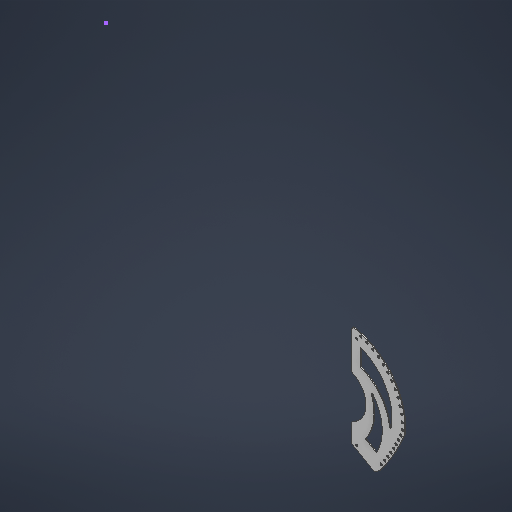
# Autodesk Inventor part: TopCurve
Saved by Autodesk Inventor 2026.1 (Build 301233000, 233)
## iProperties
Created: 2026-03-09
Part Number: TopCurve
Material: Generic
Document SubType Name: Modeling
Designer: roejo
Density: 1 g/cm^3
Appearance: Default
Author: roejo
Autodesk Inventor part; units mm, degrees
ref_plane "YZ Plane" through (0, 0, 0) normal (1, 0, 0) x (0, 1, 0)
ref_plane "XZ Plane" through (0, 0, 0) normal (0, 1, 0) x (-1, 0, 0)
ref_plane "XY Plane" through (0, 0, 0) normal (0, 0, 1) x (1, 0, 0)
sketch "Sketch1" plane through (0, 0, 0) normal (0, 0, 1) x (1, 0, 0)
  circle A0 centre (241.6154, -140.1465) radius 2.4638
  arc A1 (259.0779, -181.0227) -> (259.0779, -99.2703) centre (241.6154, -140.1465) ccw
  line L0 (259.0779, -218.2466) -> (259.0779, -181.0227)
  arc A2 (312.3724, -235.9031) -> (359.2204, -154.9095) centre (11.2573, -7.6879) ccw
  arc A3 (359.2204, -154.9095) -> (360.17, -151.1328) centre (347.5241, -149.9609) ccw
  arc A4 (360.17, -151.1328) -> (262.8183, -22.9871) centre (241.6154, -140.1465) ccw
  arc A5 (301.8563, -242.8447) -> (312.3724, -235.9031) centre (241.6154, -140.1465) ccw
  arc A6 (262.8183, -22.9871) -> (259.0779, -26.1114) centre (262.2529, -26.1114) ccw
  line L1 (259.0779, -26.1114) -> (259.0779, -99.2703)
  line L2 (259.0779, -181.0227) -> (259.0779, -218.2466)
  circle A7 centre (268.2854, -38.5465) radius 2.1844
  circle A8 centre (268.2854, -216.3465) radius 2.1844
  arc A9 (308.9934, -232.4758) -> (354.8343, -153.0538) centre (11.2573, -7.6879) ccw
  arc A10 (354.8343, -153.0538) -> (355.4278, -150.6933) centre (347.5241, -149.9609) ccw
  arc A11 (355.4278, -150.6933) -> (263.8404, -28.0281) centre (241.6154, -140.1465) ccw
  circle A12 centre (263.8404, -28.0281) radius 2.413
  circle A13 centre (276.0241, -31.1486) radius 2.413
  circle A14 centre (287.7911, -35.5889) radius 2.413
  circle A15 centre (298.9991, -41.2951) radius 2.413
  circle A16 centre (309.5123, -48.1981) radius 2.413
  circle A17 centre (319.2034, -56.2144) radius 2.413
  circle A18 centre (327.9551, -65.247) radius 2.413
  circle A19 centre (335.6615, -75.1863) radius 2.413
  circle A20 centre (342.2292, -85.9122) radius 2.413
  circle A21 centre (347.5787, -97.2948) radius 2.413
  circle A22 centre (351.6452, -109.1961) radius 2.413
  circle A23 centre (354.3796, -121.4722) radius 2.413
  circle A24 centre (355.7487, -133.9744) radius 2.413
  circle A25 centre (355.7358, -146.5513) radius 2.413
  circle A26 centre (353.0365, -157.2317) radius 2.413
  circle A27 centre (348.7088, -166.7567) radius 2.413
  circle A28 centre (344.0523, -176.2817) radius 2.413
  circle A29 centre (339.0531, -185.8067) radius 2.413
  circle A30 centre (333.6952, -195.3317) radius 2.413
  circle A31 centre (327.9604, -204.8567) radius 2.413
  circle A32 centre (321.8278, -214.3817) radius 2.413
  circle A33 centre (315.2734, -223.9067) radius 2.413
  line L3 (301.8563, -242.8447) -> (259.0779, -218.2466)
  point P0 (259.0779, -22.3716)
  point P1 (295.3179, -246.41)
  dimension "d4" = 88.9
  dimension "d5" = 12.7
  dimension "d7" = 4.3688
  dimension "d8" = 4.7625
  dimension "d9" = 4.826
  dimension "d12" = 82
  dimension "d14" = 4.826
  dimension "d21" = 4.826
  dimension "d22" = 4.826
  dimension "d23" = 4.826
  dimension "d24" = 4.826
  dimension "d25" = 4.826
  dimension "d26" = 4.826
  dimension "d27" = 4.826
  dimension "d28" = 9.525
  dimension "d29" = 9.525
  dimension "d30" = 9.525
  dimension "d31" = 9.525
  dimension "d32" = 9.525
  dimension "d33" = 9.525
  dimension "d34" = 9.525
  dimension "d41" = 177.8
  dimension "d42" = 9.2075
  constraints: 33 centre point, 18 point on circle, 8 end point, 4 tangent, 3 coincident, 45 other
  measures "d4" diameter of A1
  measures "d5" radius of A3
  measures "d7" diameter of A8
  measures "d8" radial gap between concentric circles of A4 A11
  measures "d9" diameter of A12
  measures "d14" diameter of A26
  measures "d21" diameter of A27
  measures "d22" diameter of A28
  measures "d23" diameter of A29
  measures "d24" diameter of A30
  measures "d25" diameter of A31
  measures "d26" diameter of A32
  measures "d27" diameter of A33
  measures "d28" vertical distance of A27.centre A26.centre
  measures "d29" vertical distance of A28.centre A27.centre
  measures "d30" vertical distance of A29.centre A28.centre
  measures "d31" vertical distance of A30.centre A29.centre
  measures "d32" vertical distance of A31.centre A30.centre
  measures "d33" vertical distance of A32.centre A31.centre
  measures "d34" vertical distance of A32.centre A33.centre
  measures "d41" distance of A8.centre A7.centre
  measures "d42" distance from line of L1 A7.centre
extrude "Extrusion1" add sketch "Sketch1" along normal blind 1.5875 contours A1 L1 A6 A4 A3 A2 A5 L3 L0
sketch "Sketch4" plane through (0, 0, 1.5875) normal (0, 0, 1) x (1, 0, 0)
  point P0 (-212.5628, 245.6595)
sketch "Sketch6" plane through (0, 0, 1.5875) normal (0, 0, 1) x (1, 0, 0)
  circle A0 centre (263.8404, -28.0281) radius 2.413 projected
  point P0 (0, 0)
extrude "Extrusion4" add sketch "Sketch6" against normal blind 1.5875
sketch "Sketch7" plane through (0, 0, 1.5875) normal (0, 0, 1) x (1, 0, 0)
  arc A0 (259.0779, -181.0227) -> (259.0779, -99.2703) centre (241.6154, -140.1465) ccw projected
  arc A1 (360.17, -151.1328) -> (262.8183, -22.9871) centre (241.6154, -140.1465) ccw projected
  arc A2 (359.2204, -154.9095) -> (360.17, -151.1328) centre (347.5241, -149.9609) ccw projected
  arc A3 (312.3724, -235.9031) -> (359.2204, -154.9095) centre (11.2573, -7.6879) ccw projected
  arc A4 (301.8563, -242.8447) -> (312.3724, -235.9031) centre (241.6154, -140.1465) ccw projected
  line L0 (259.0779, -218.2466) -> (301.8563, -242.8447) projected
  line L1 (259.0779, -181.0227) -> (259.0779, -218.2466) projected
  line L2 (259.0779, -26.1114) -> (259.0779, -99.2703) projected
  arc A5 (262.8183, -22.9871) -> (259.0779, -26.1114) centre (262.2529, -26.1114) ccw projected
  arc A6 (306.6939, -207.6622) -> (299.0406, -115.0702) centre (233.6747, -167.0854) ccw
  line L3 (304.5149, -208.2673) -> (286.208, -197.7406)
  arc A7 (285.7036, -195.4472) -> (296.3064, -116.6011) centre (215.7134, -145.8993) ccw
  arc A8 (331.0433, -153.7665) -> (275.984, -82.4202) centre (246.0316, -162.4533) ccw
  arc A9 (334.1816, -153.9043) -> (277.1253, -49.9392) centre (242.868, -136.3786) ccw
  arc A10 (331.0433, -153.7665) -> (334.1816, -153.9043) centre (332.6226, -153.6051) ccw
  arc A11 (299.0406, -115.0702) -> (296.3064, -116.6011) centre (297.7984, -116.0587) ccw
  line L4 (274.9529, -51.4151) -> (274.9529, -80.9334)
  arc A12 (277.1253, -49.9392) -> (274.9529, -51.4151) centre (276.5404, -51.4151) ccw
  arc A13 (274.9529, -80.9334) -> (275.984, -82.4202) centre (276.5404, -80.9334) ccw
  arc A14 (285.7036, -195.4472) -> (286.208, -197.7406) centre (286.9993, -196.3644) ccw
  arc A15 (304.5149, -208.2673) -> (306.6939, -207.6622) centre (305.3062, -206.8911) ccw
  point P0 (0, 0)
  point P1 (305.8979, -209.0626)
  point P2 (284.6802, -196.8621)
  point P3 (274.9529, -82.0418)
  point P4 (274.9529, -49.1096)
  dimension "d51" = 1.5875
  dimension "d52" = 1.5875
  constraints: 24 point on circle, 12 tangent, 10 centre point, 4 end point, 4 equal radius, 4 point on line, 1 vertical
  measures "d51" radius of A10
  measures "d52" radius of A12
extrude "Extrusion5" cut sketch "Sketch7" against normal blind 1.5875 contours A15 L3 A14 A7 A11 A6 | A8 A13 L4 A12 A9 A10
body "Solid1"
